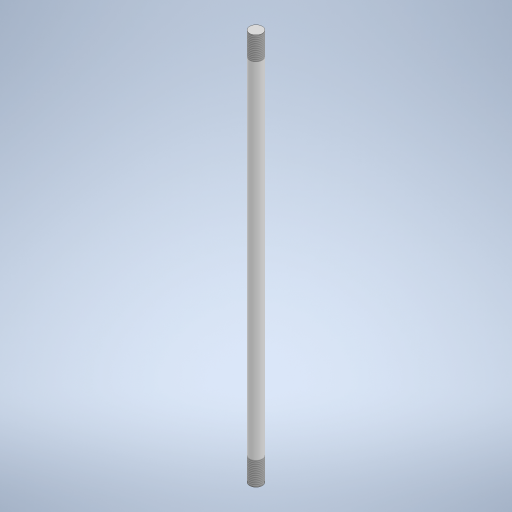
# Autodesk Inventor part: oś
Saved by Autodesk Inventor 2024 (Build 280153000, 153)
## iProperties
Created: 2024-11-28
Part Number: oś
Material: Ogólny
Document SubType Name: Modeling
Designer: fkoba.i_ekonomik
Density: 1 g/cm^3
Appearance: Domyślna
Author: fkoba.i_ekonomik
Autodesk Inventor part; units mm, degrees
ref_plane "YZ Plane" through (0, 0, 0) normal (1, 0, 0) x (0, 1, 0)
ref_plane "XZ Plane" through (0, 0, 0) normal (0, 1, 0) x (-1, 0, 0)
ref_plane "XY Plane" through (0, 0, 0) normal (0, 0, 1) x (1, 0, 0)
sketch "Szkic1" plane through (0, 0, 0) normal (0, 1, 0) x (-1, 0, 0)
  circle A0 centre (0, 0) radius 8
  dimension "d0" = 16
  constraints: 1 centre point, 1 coincident
  measures "d0" diameter of A0
extrude "Wyciągnięcie proste1" add sketch "Szkic1" along normal blind 250
thread "Gwint1" size "M16x2" class "6g" standard "ANSI Metric M Profile" length 30
mirror "Odbij1" about plane through (0, 250, 0) normal (0, 1, 0)
